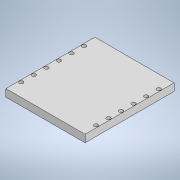
# Autodesk Inventor part: Драйвер моторов DRV8833
Saved by Autodesk Inventor 2020 (Build 240168000, 168)
## iProperties
Created: 2021-08-09
Part Number: Драйвер моторов DRV8833
Material: Типовые
Document SubType Name: Modeling
Designer: Антон
Density: 1 g/cm^3
Appearance: По умолчанию
Author: Антон
Autodesk Inventor part; units mm, degrees
ref_plane "YZ Plane" through (0, 0, 0) normal (1, 0, 0) x (0, 1, 0)
ref_plane "XZ Plane" through (0, 0, 0) normal (0, 1, 0) x (-1, 0, 0)
ref_plane "XY Plane" through (0, 0, 0) normal (0, 0, 1) x (1, 0, 0)
sketch "Эскиз1" plane through (0, 0, 0) normal (0, 1, 0) x (-1, 0, 0)
  line L0 (0, 0) -> (16, 0)
  line L1 (16, 0) -> (16, -18)
  line L2 (16, -18) -> (0, -18)
  line L3 (0, -18) -> (0, 0)
  dimension "d0" = 16
  dimension "d1" = 18
  constraints: 8 end point, 2 parallel, 1 horizontal, 1 perpendicular
  measures "d0" distance of L1.end L2.end
  measures "d1" distance of L0.end L1.end
extrude "Выдавливание1" add sketch "Эскиз1" along normal blind 1.5
sketch "Эскиз2" plane through (0, 1.5, 0) normal (0, 1, 0) x (1, 0, 0)
  line L0 (-16, 18) -> (-16, 0) projected
  line L1 (-16, 0) -> (0, 0) construction
  line L2 (-8, 0) -> (-8, 18) construction
  line L3 (0, 18) -> (-16, 18) construction
  line L4 (-15.56, 2.65) -> (-15.56, 0) construction
  line L5 (-15.56, 15.35) -> (-15.56, 18) construction
  line L6 (-15.56, 2.65) -> (-16, 2.65) construction
  point P0 (-15.56, 12.81)
  point P1 (-15.56, 10.27)
  point P2 (-15.56, 7.73)
  point P3 (-15.56, 5.19)
  point P4 (-0.44, 15.35)
  point P5 (-0.44, 12.81)
  point P6 (-0.44, 10.27)
  point P7 (-0.44, 7.73)
  point P8 (-0.44, 5.19)
  point P9 (-0.44, 2.65)
  dimension "d6" = 2.54
  dimension "d11" = 15.12
  constraints: 8 end point, 6 symmetric about line, 3 point on line, 2 midpoint, 2 perpendicular, 2 vertical, 1 collinear, 5 other
  measures "d6" distance of L5.start point (-15.56, 12.81)
  measures "d11" distance of point (-0.44, 2.65) L4.start
hole "Отверстие1" at (-15.56, 1.5, -15.35) at (-15.56, 1.5, -12.81) at (-15.56, 1.5, -10.27) at (-15.56, 1.5, -7.73) at (-15.56, 1.5, -5.19) at (-15.56, 1.5, -2.65) at (-0.44, 1.5, -2.65) at (-0.44, 1.5, -5.19) at (-0.44, 1.5, -7.73) at (-0.44, 1.5, -10.27) at (-0.44, 1.5, -12.81) at (-0.44, 1.5, -15.35) direction (0, -1, 0) diameter 0.8 end through all
